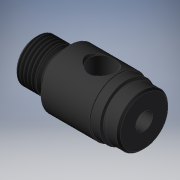
# Autodesk Inventor part: 0.75DXP-H_SRS1
Saved by Autodesk Inventor 2019 (Build 230136000, 136)
## iProperties
Created: 2023-02-15
Part Number: 0.75DXP-H_SRS1
Material: Generic
Catalog Web Link: www.cadenas.de
Description: SR Series Head-Pneumatic Cylinder
Vendor: PARKERHANNIFIN
Document SubType Name: Modeling
Designer: psAdmin
Manufacturer: PARKERHANNIFIN
Mass: 10.1254 g
Surface Area: 41.2397 cm^2
Volume: 10.1254 cm^3
Density: 1 g/cm^3
Appearance: PSOLRGB-175-175-175
Category: PARTsolutions
Company: PARKERHANNIFIN
Title: 0.75DXP-H_SRS1
Author: Cadenas PARTsolutions
Comments: Pneumatic Cylinder
PSOL_IDENT_0: {$CADENAS_DATA/23d-libs/parkerpdn/actuators_cylinders/pneumatic_cylinders/sr_series/parts/sr_head_ca
PSOL_IDENT_1: p.prj},207 {VTYP=3D},{NB=0.75DXP-H_SRS1},{LINA=0.75DXP-H_SRS1},{NN=SR Series Head},{DATE=26.07.2021
PSOL_IDENT_2: 05:25:39},{GEOMDATE=25.09.2019 05:53:45},{VERSION=},{LINEID=40},{WBVAR=MNT,USE,CUH,SPEC,PL,SER,NL,RR
PSOL_IDENT_3: PT},{WBNUMERIC=}  {NB=0.75DXP-H_SRS1},{LINA=0.75DXP-H_SRS1},{KT=DUMMY},{PN=0.75DXP-H_SR},{BORE=0.750
PSOL_IDENT_4: 0},{BORECON=0.7500},{MNT=DXP},{MNTALG= 'N' , 'N - Nose Mount, Spring Return' , 'NR' , 'NR - Nose Mou
PSOL_IDENT_5: nt, Spring Return, Hex Rod (non-rotating)' , 'NRP' , 'NRP - Pivot and Nose Mount, Spring Return, Hex
PSOL_IDENT_6: Rod (non-rotating)' , 'P' , 'P - Pivot Mount, Spring Return' , 'R' , 'R - Nose Mount, Spring Extend
PSOL_IDENT_7: ed' , 'RP' , 'RP - Pivot and Nose Mount, Spring Extend' , 'D' , 'D - Nose Mount, Double Acting','DP'
PSOL_IDENT_8: , 'DP - Pivot and Nose Mount, Double Acting, Pivot Pin' , 'DXP' , 'DXP - Pivot and Nose Mount, Doub
PSOL_IDENT_9: le Acting, No Pivot Pin' , 'DX' , 'DX - Threaded Both End, Double Acting' ,  'A' , 'A - Nose Mount,
PSOL_IDENT_10: Spring Return, Head Adjustable Stroke' , 'RA' , 'RA - Nose Mount, Spring Extend, Cap Adjustable Stro
PSOL_IDENT_11: ke' , 'AP' , 'AP - Pivot Mount, Spring Return, Head Adjustable Stroke' , 'AR' , 'AR - Air Reservoirs'
PSOL_IDENT_12: , 'BRN' , 'BRN - Rear Block Mount, Single Acting' , 'BRR' , 'BRR - Rear Block Mount, Single Acting,
PSOL_IDENT_13: Spring Return' , 'BFD' , 'BFD - Front Block Mount, Double Acting' , 'BRD' , 'BRD - Rear Block Mount
PSOL_IDENT_14: , Double Acting' , 'BFN' , 'BFN - Front Block Mount, Single Acting, Spring Return' , 'BFR' , 'BFR -
PSOL_IDENT_15: Front Block Mount, Single Acting, Spring Extend' , 'TRN' , 'TRN - Rear Trunnion Mount, Single Acting
PSOL_IDENT_16: , Spring Return' , 'TRR' , 'TRR - Rear Trunnion Mount, Single Acting, Spring Extend' , 'TFD' , 'TFD
PSOL_IDENT_17: - Front Trunnion Mount, Double Acting' , 'TRD' , 'TRD - Rear Trunnion Mount, Double Acting' , 'TFN'
PSOL_IDENT_18: , 'TFN - Front Trunnion Mount, Single Acting, Spring Return' , 'TFR' , 'TFR - Front Trunnion Mount,
PSOL_IDENT_19: Single Acting, Spring Extend' },{USE=H},{USEALG=  'H', 'Head', 'C', 'Cap' },{CUH=},{CUHALG= '' , 'No
PSOL_IDENT_20: Cushion' , 'C' , 'C - Cushion' },{SPEC=S},{PL=1},{THD=0.6250},{THD1=0.5000},{THD2=0.5000},{THD3=0.6
PSOL_IDENT_21: 250},{TAB=UNF},{L=1.59500},{OD=0.85500},{SQ=0.00000},{SQW=0.00000},{THDLEN=0.32000},{L1=1.09300},{L2=
PSOL_IDENT_22: 0.38000},{L3=0.25000},{L31=0.18800},{L4=0.03600},{D1=0.70100},{D2=0.75800},{D3=0.00000},{D4=0.81500}
PSOL_IDENT_23: ,{C1=0.03000},{CC=0.25000},{PD=0.37500},{PLHELP=1},{ROT=-90},{EETHD=0.40500},{EETHD1=0.40500},{EETAB=
PSOL_IDENT_24: NPTF},{CBOREDEP=0.00000},{CBOREDIA=0.00000},{HEX=0.00000},{HEXDEP=0.00000},{XW=0.00000},{XD=0.00000}
PSOL_IDENT_25: ,{TD=0.50000},{TL=0.37500},{TRDIS=0.35000},{TRDIS1=0.35000},{TRDIS2=0.37000},{DA=0.00000},{DADEP=0.0
PSOL_IDENT_26: 0000},{DB=0.00000},{CF=0.00000},{CP=0.00000},{HP=0.62500},{FH=0.37500},{BC=1.00000},{S=0.19000},{SDE
PSOL_IDENT_27: P=0.34400},{STAB=UNF},{ASTHD=0.43750},{SO=0.25000},{SODEP=0.50000},{SC=0.33300},{SCDEP=0.20800},{CL1=
PSOL_IDENT_28: 0.08200},{CL2=0.10000},{CD1=0.62200},{CD2=0.53700},{CR1=0.03000},{CUX=0.62500},{CUY=0.25900},{CUD1=0
PSOL_IDENT_29: .22800},{CUD2=0.16100},{FOD=0.34300},{CUD2DEP=0.15600},{CUTHD=3.000},{PCUT=0.00000},{PCUT1=0.37000},
PSOL_IDENT_30: {PCUT2=0.00000},{PCUTDEP=0.00800},{PDIA=0.25150},{PDIA1=0.25150},{PDIA2=0.25000},{PDIA3=0.31400},{PD
PSOL_IDENT_31: IS=1.07000},{PDIS1=1.07000},{WC=0.00000},{WCDEP=0.18800},{NOTHD=0},{LENGTH=1.34500},{NUTCON=0.625},{
PSOL_IDENT_32: OLEN=1.59500},{BUSH=0},{SER=SR},{PLCALG='None','None','1','Port Position 1 Cap End','2','Port Positi
PSOL_IDENT_33: on 2 Cap End','3','Port Position 3 Cap End','4','Port Position 4 Cap End'},{PLHELP1=1},{NL=},{ROTCUH=
PSOL_IDENT_34: 0.000},{NLALG='','N/A'},{RRPT=},{RRPTALG= '','N/A' }
NB: 0.75DXP-H_SRS1
NN: SR Series Head
NT: Pneumatic Cylinder
NBSYN: $PN.$SPEC.$PL.$NL.$RRPT.
LINA: 0.75DXP-H_SRS1
CATALOG: Parker Pneumatic Division
BORE: 0.75
BORECON: 0.7500
MNT: DXP - Pivot and Nose Mount, Double Acting, No Pivot Pin
USE: Head
CUH: No Cushion
SPEC: Special Modifications
PL: Port Position 1 Cap End
THD1: 0.5
THD2: 0.5
THD3: 0.625
TAB: UNF
L31: 0.188
L4: 0.036
D1: 0.701
D2: 0.758
C1: 0.03
CC: 0.25
EETHD1: 0.405
EETAB: NPTF
TD: 0.5
TL: 0.375
TRDIS1: 0.35
TRDIS2: 0.37
DA: 0
DADEP: 0
DB: 0
CF: 0
CP: 0
HP: 0.625
FH: 0.375
BC: 1
S: 0.19
SDEP: 0.344
STAB: UNF
ASTHD: 0.4375
SO: 0.25
SODEP: 0.5
SC: 0.333
SCDEP: 0.208
CL1: 0.082
CR1: 0.03
CUX: 0.625
CUY: 0.259
CUD1: 0.228
CUD2: 0.161
FOD: 0.343
CUD2DEP: 0.156
CUTHD: 3
PCUT1: 0.37
PCUT2: 0
PCUTDEP: 0.008
PDIA1: 0.2515
PDIA2: 0.25
PDIA3: 0.314
PDIS1: 1.07
WCDEP: 0.188
SER: SR
NL: N/A
RRPT: N/A
SUPPLIER: PARKERHANNIFIN
ARTICLENO: 0.75DXP-H_SRS1
BOMINFO: 0.75DXP-H_SRS1
CREATOR: CADENAS GmbH
Autodesk Inventor part; units mm, degrees
sketch "Sketch_1" plane through (0, 0, 0) normal (0, 0, 1) x (1, 0, 0)
  line L0 (18.1102, 0) -> (0, 0)
  line L1 (0, 0) -> (0, 10.8585)
  line L2 (0, 10.8585) -> (18.1102, 10.8585)
  line L3 (18.1102, 10.8585) -> (18.1102, 0)
  line L4 (18.1102, 0) -> (0, 0)
  constraints: 10 end point
revolve "Revolution1" add sketch "Sketch_1" angle 360 about axis through (18.1102, 0, 0) along (1, 0, 0)
sketch "Sketch_2" plane through (0, 0, 0) normal (0, 0, 1) x (1, 0, 0)
  line L0 (0, 0) -> (-12.7508, 0)
  line L1 (-12.7508, 0) -> (-12.7508, 7.098)
  line L2 (-12.7508, 7.098) -> (-11.9113, 7.9375)
  line L3 (-11.9113, 7.9375) -> (0, 7.9375)
  line L4 (0, 7.9375) -> (0, 0)
  line L5 (0, 0) -> (-12.7508, 0)
  constraints: 12 end point
revolve "Revolution2" add sketch "Sketch_2" angle 360 about axis through (0, 0, 0) along (1, 0, 0)
thread "Thread1" size "5/8-18 UNF" class "2A" standard "ANSI Unified Screw Threads" length 7.2885
sketch "Sketch_6" plane through (0, 0, 0) normal (0, 0, 1) x (1, 0, 0)
  line L0 (27.7622, 0) -> (18.1102, 0)
  line L1 (18.1102, 0) -> (18.1102, 10.3505)
  line L2 (18.1102, 10.3505) -> (21.4122, 10.3505)
  line L3 (21.4122, 10.3505) -> (21.4122, 8.9027)
  line L4 (21.4122, 8.9027) -> (22.3266, 8.9027)
  line L5 (22.3266, 8.9027) -> (23.0505, 9.6266)
  line L6 (23.0505, 9.6266) -> (27.0002, 9.6266)
  line L7 (27.0002, 9.6266) -> (27.7622, 8.8646)
  line L8 (27.7622, 8.8646) -> (27.7622, 0)
  line L9 (27.7622, 0) -> (18.1102, 0)
  constraints: 20 end point
revolve "Revolution3" add sketch "Sketch_6" angle 360 about axis through (27.7622, 0, 0) along (1, 0, 0)
sketch "Sketch_7" plane through (0, 0, 0) normal (1, 0, 0) x (0, 1, 0)
  circle A0 centre (0, 0) radius 3.175
  constraints: 1 centre point
extrude "Extrusion1" cut sketch "Sketch_7" along normal mid plane 111.0488
sketch "Sketch_8" plane through (11.8872, 0, 0) normal (0, 0, 1) x (0, -1, 0)
  line L0 (0, 0) -> (-11.7085, 0)
  line L1 (-11.7085, 0) -> (-11.7085, 6.4547)
  line L2 (-11.7085, 6.4547) -> (-10.0692, 4.8153)
  line L3 (-10.0692, 4.8153) -> (0, 4.501)
  line L4 (0, 4.501) -> (0, 0)
  line L5 (0, 0) -> (-11.7085, 0)
  constraints: 12 end point
revolve "Revolution4" cut sketch "Sketch_8" angle 360 about axis through (11.8872, 0, 0) along (0, -1, 0)
sketch "Sketch_29" plane through (0, 0, 0) normal (0, 0, 1) x (1, 0, 0)
  line L0 (0, 0) -> (-4.6228, 0)
  line L1 (-4.6228, 9.8994) -> (-4.6228, 7.9375)
  line L2 (-4.6228, 7.9375) -> (-3.7284, 7.0431)
  arc A0 (-3.7284, 7.0431) -> (-3.1896, 6.8199) centre (-3.1896, 7.5819) ccw
  line L3 (-3.1896, 6.8199) -> (-2.7567, 6.8199)
  arc A1 (-2.7567, 6.8199) -> (-2.0828, 7.2263) centre (-2.7567, 7.5819) ccw
  line L4 (-2.0828, 7.2263) -> (-2.0828, 7.8994)
  line L5 (-2.0828, 7.8994) -> (0, 7.8994)
  line L6 (0, 7.8994) -> (0, 9.8994)
  line L7 (0, 9.8994) -> (-4.6228, 9.8994)
  constraints: 16 end point, 4 point on circle, 2 centre point
revolve "Revolution5" cut sketch "Sketch_29" angle 360 about axis through (0, 0, 0) along (1, 0, 0)
ref_plane "b1_XY" through (0, 7.8994, 0) normal (1, 0, 0) x (0, 0, -1)
ref_plane "b1_YZ" through (0, 7.8994, 0) normal (0, 0, -1) x (0, 1, 0)
ref_plane "b1_ZX" through (0, 7.8994, 0) normal (0, 1, 0) x (1, 0, 0)
ref_plane "b2_XY" through (0, -7.8994, 0) normal (1, 0, 0) x (0, 0, -1)
ref_plane "b2_YZ" through (0, -7.8994, 0) normal (0, 0, -1) x (0, 1, 0)
ref_plane "b2_ZX" through (0, -7.8994, 0) normal (0, 1, 0) x (1, 0, 0)
ref_plane "cl1_XY" through (0, 0, 0) normal (0, 0, 1) x (1, 0, 0)
ref_plane "cl1_YZ" through (0, 0, 0) normal (1, 0, 0) x (0, 1, 0)
ref_plane "cl1_ZX" through (0, 0, 0) normal (0, 1, 0) x (0, 0, 1)
ref_plane "cl2_XY" through (-2.0828, 0, 0) normal (0, 0, 1) x (1, 0, 0)
ref_plane "cl2_YZ" through (-2.0828, 0, 0) normal (1, 0, 0) x (0, 1, 0)
ref_plane "cl2_ZX" through (-2.0828, 0, 0) normal (0, 1, 0) x (0, 0, 1)
ref_plane "ee_XY" through (11.8872, 10.8585, 0) normal (1, 0, 0) x (0, -1, 0)
ref_plane "ee_YZ" through (11.8872, 10.8585, 0) normal (0, -1, 0) x (0, 0, -1)
ref_plane "ee_ZX" through (11.8872, 10.8585, 0) normal (0, 0, -1) x (1, 0, 0)
ref_plane "od1_XY" through (0, 0, 10.8585) normal (1, 0, 0) x (0, 0, -1)
ref_plane "od1_YZ" through (0, 0, 10.8585) normal (0, 0, -1) x (0, 1, 0)
ref_plane "od1_ZX" through (0, 0, 10.8585) normal (0, 1, 0) x (1, 0, 0)
ref_plane "od2_XY" through (0, 0, -10.8585) normal (1, 0, 0) x (0, 0, -1)
ref_plane "od2_YZ" through (0, 0, -10.8585) normal (0, 0, -1) x (0, 1, 0)
ref_plane "od2_ZX" through (0, 0, -10.8585) normal (0, 1, 0) x (1, 0, 0)
ref_plane "od3_XY" through (0, 10.8585, 0) normal (1, 0, 0) x (0, 0, -1)
ref_plane "od3_YZ" through (0, 10.8585, 0) normal (0, 0, -1) x (0, 1, 0)
ref_plane "od3_ZX" through (0, 10.8585, 0) normal (0, 1, 0) x (1, 0, 0)
ref_plane "od4_XY" through (0, -10.8585, 0) normal (1, 0, 0) x (0, 0, -1)
ref_plane "od4_YZ" through (0, -10.8585, 0) normal (0, 0, -1) x (0, 1, 0)
ref_plane "od4_ZX" through (0, -10.8585, 0) normal (0, 1, 0) x (1, 0, 0)
ref_plane "to_body_XY" through (21.4122, 0, 0) normal (1, 0, 0) x (0, 0, -1)
ref_plane "to_body_YZ" through (21.4122, 0, 0) normal (0, 0, -1) x (0, 1, 0)
ref_plane "to_body_ZX" through (21.4122, 0, 0) normal (0, 1, 0) x (1, 0, 0)
ref_plane "to_dummy_XY" through (0, 0, 0) normal (1, 0, 0) x (0, 0, -1)
ref_plane "to_dummy_YZ" through (0, 0, 0) normal (0, 0, -1) x (0, 1, 0)
ref_plane "to_dummy_ZX" through (0, 0, 0) normal (0, 1, 0) x (1, 0, 0)
ref_plane "to_nut_XY" through (-12.7508, 0, 0) normal (1, 0, 0) x (0, 0, -1)
ref_plane "to_nut_YZ" through (-12.7508, 0, 0) normal (0, 0, -1) x (0, 1, 0)
ref_plane "to_nut_ZX" through (-12.7508, 0, 0) normal (0, 1, 0) x (1, 0, 0)
ref_plane "to_stroke_adjuster_XY" through (27.7622, 0, 0) normal (1, 0, 0) x (0, 0, -1)
ref_plane "to_stroke_adjuster_YZ" through (27.7622, 0, 0) normal (0, 0, -1) x (0, 1, 0)
ref_plane "to_stroke_adjuster_ZX" through (27.7622, 0, 0) normal (0, 1, 0) x (1, 0, 0)
body "Solid1"
